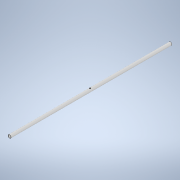
# Autodesk Inventor part: horizontal support
Saved by Autodesk Inventor 2021 (Build 250183000, 183)
## iProperties
Created: 2020-07-11
Part Number: horizontal support
Material: Generic
Document SubType Name: Modeling
Designer: Shannon
Density: 1 g/cm^3
Appearance: Default
Author: Shannon
Autodesk Inventor part; units mm, degrees
ref_plane "YZ Plane" through (0, 0, 0) normal (1, 0, 0) x (0, 1, 0)
ref_plane "XY Plane" through (0, 0, 0) normal (0, 0, 1) x (1, 0, 0)
sketch "Sketch1" plane through (0, 0, 0) normal (0, 0, 1) x (1, 0, 0)
  circle A0 centre (0, 0) radius 6.35
  dimension "d0" = 12.7
  constraints: 1 centre point, 1 coincident
  measures "d0" diameter of A0
extrude "Extrusion1" add sketch "Sketch1" along normal blind 660.4
sketch "Sketch2" plane through (0, 0, 660.4) normal (0, 0, 1) x (1, 0, 0)
  circle A0 centre (0, 0) radius 5.334
  dimension "d3" = 10.668
  constraints: 1 centre point, 1 coincident
  measures "d3" diameter of A0
extrude "Extrusion2" cut sketch "Sketch2" against normal blind 660.4
ref_plane "Work Plane1" through (0, 6.35, 0) normal (0, 1, 0) x (-1, 0, 0)
sketch "Sketch3" plane through (0, 6.35, 0) normal (0, 1, 0) x (-1, 0, 0)
  circle A0 centre (0, 330.2) radius 2.8654
  point P0 (0, 0)
  dimension "d6" = 330.2
  constraints: 1 centre point
  measures "d6" distance of point (0, 0) A0.centre
extrude "Extrusion3" cut sketch "Sketch3" against normal through all
body "Solid1"
